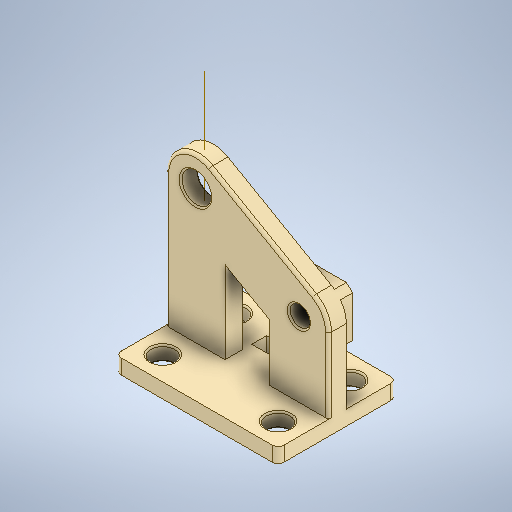
# Autodesk Inventor part: Steering Mounting Plate
Saved by Autodesk Inventor 2025.2 (Build 292293000, 293)
## iProperties
Created: 2025-02-04
Part Number: Steering Mounting Plate
Material: Generic
Document SubType Name: Modeling
Designer: eason
Density: 1 g/cm^3
Appearance: Beige
Author: eason
Autodesk Inventor part; units mm, degrees
ref_plane "YZ Plane" through (0, 0, 0) normal (1, 0, 0) x (0, 1, 0)
ref_plane "XZ Plane" through (0, 0, 0) normal (0, 1, 0) x (-1, 0, 0)
ref_plane "XY Plane" through (0, 0, 0) normal (0, 0, 1) x (1, 0, 0)
sketch "Sketch1" plane through (0, 0, 0) normal (0, 0, 1) x (1, 0, 0)
  circle A0 centre (0, 0) radius 5
  line L0 (44.8948, -50) -> (-10, -50)
  line L1 (-10, -50) -> (-10, 0)
  line L2 (0, 5) -> (-5, 5) construction
  line L3 (-5, 5) -> (-5, 0) construction
  line L4 (-10, -50) -> (44.8948, -50)
  line L5 (44.8948, -45) -> (-10, -45)
  line L6 (-10, -45) -> (-10, -50)
  line L7 (0, 0) -> (34.8948, -20) construction
  circle A1 centre (34.8948, -20) radius 3.4
  arc A2 (4.9727, 8.676) -> (-10, 0) centre (0, 0) ccw
  line L8 (-24.2121, 0) -> (57.773, 0) projected
  arc A3 (44.8948, -20) -> (39.8675, -11.324) centre (34.8948, -20) ccw
  line L9 (44.8948, -20) -> (44.8948, -50)
  line L10 (4.9727, 8.676) -> (39.8675, -11.324)
  line L11 (10, -17.2576) -> (24.8948, -25.7946)
  line L12 (24.8948, -25.7946) -> (24.8948, -45)
  line L13 (10, -17.2576) -> (10, -45)
  point P0 (-10, -45)
  dimension "d2" = 10
  dimension "d5" = 5
  dimension "d7" = 5
  dimension "d47" = 40.22
  dimension "d48" = 6.8
  dimension "d50" = 25
  dimension "d51" = 20
  dimension "d53" = 45
  constraints: 27 end point, 10 tangent, 6 point on circle, 4 centre point, 4 coincident, 4 point on line, 3 perpendicular, 2 horizontal, 1 parallel
  measures "d2" diameter of A0
  measures "d5" distance between parallel lines of L1 L3
  measures "d7" distance between parallel lines of L0 L5
  measures "d47" distance of L7.start L7.end
  measures "d48" diameter of A1
  measures "d50" distance from line of L5 L7.end
  measures "d51" diameter of A3
  measures "d53" distance from line of L5 L7.start
extrude "Extrusion1" add sketch "Sketch1" along normal mid plane 6 contours L8 L10 A3 L9 L5 L12 L11 L13 L1 A0 | A0 L8 A2 L10
extrude "Extrusion2" add sketch "Sketch1" along normal mid plane 40 contours L5 L9 L0 L1
sketch "Sketch2" plane through (-10, -50, 20) normal (0, -1, 0) x (1, 0, 0)
  circle A0 centre (46.8948, -32) radius 4
  circle A1 centre (46.8948, -8) radius 4
  circle A2 centre (8, -32) radius 4
  circle A3 centre (8, -8) radius 4
  line L0 (54.8948, -40) -> (0, -40) projected
  line L1 (54.8948, 0) -> (54.8948, -40) projected
  line L2 (0, 0) -> (54.8948, 0) projected
  line L3 (0, -40) -> (0, 0) projected
  point P0 (10, -20)
  dimension "d14" = 8
  dimension "d15" = 8
  dimension "d16" = 8
  dimension "d17" = 8
  dimension "d18" = 8
  dimension "d19" = 8
  dimension "d20" = 8
  dimension "d21" = 8
  dimension "d22" = 8
  dimension "d23" = 8
  dimension "d24" = 8
  dimension "d25" = 8
  constraints: 4 centre point
  measures "d14" diameter of A0
  measures "d15" diameter of A1
  measures "d16" diameter of A2
  measures "d17" diameter of A3
  measures "d18" distance from line of L0 A0.centre
  measures "d19" distance from line of L1 A0.centre
  measures "d20" distance from line of L2 A1.centre
  measures "d21" distance from line of L1 A1.centre
  measures "d22" distance from line of L3 A3.centre
  measures "d23" distance from line of L2 A3.centre
  measures "d24" distance from line of L0 A2.centre
  measures "d25" distance from line of L3 A2.centre
extrude "Extrusion3" cut sketch "Sketch2" against normal up to surface (5 mm away) contours A0 | A1 | A2 | A3
fillet "Fillet1" radius 2 4 edges at (-10, -47.5, -20) (-10, -47.5, 20) (44.8948, -47.5, -20) (44.8948, -47.5, 20)
fillet "Fillet2" radius 1 1 edges at (-10, -22.5, 3)
fillet "Fillet3" radius 0.5 11 edges at (-5, 0, 3) (-5, 0, -3) (-6, -45, 12) (-6, -50, 12) (32.8948, -45, 12) (32.8948, -50, 12) (32.8948, -45, -12) (32.8948, -50, -12) (-6, -45, -12) (-6, -50, -12) (31.4948, -20, 3)
sketch "Sketch3" plane through (0, 0, -3) normal (0, 0, -1) x (-1, 0, 0)
  line L0 (-40.9448, -14) -> (-28.8448, -14)
  line L1 (-28.8448, -14) -> (-28.8448, -26)
  line L2 (-28.8448, -26) -> (-40.9448, -26)
  line L3 (-40.9448, -26) -> (-40.9448, -14)
  line L4 (-40.9448, -14) -> (-28.8448, -26) construction
  line L5 (-28.8448, -14) -> (-40.9448, -26) construction
  line L6 (-26.8448, -12) -> (-26.8448, -28)
  line L7 (-26.8448, -28) -> (-42.9448, -28)
  circle A0 centre (-34.8948, -20) radius 3.4
  circle A1 centre (-34.8948, -20) radius 3.4 projected
  line L8 (-42.9448, -12.0165) -> (-42.9448, -12)
  arc A2 (-39.8675, -11.324) -> (-44.8948, -20) centre (-34.8948, -20) ccw projected
  line L9 (-42.9448, -28) -> (-42.9448, -14.0673)
  arc A3 (-39.8675, -11.324) -> (-44.8948, -20) centre (-34.8948, -20) ccw projected
  line L10 (-26.8448, -12) -> (-40.8948, -12)
  point P0 (0, 0)
  dimension "d31" = 12
  dimension "d32" = 12.1
  dimension "d35" = 2
  dimension "d36" = 2
  dimension "d54" = 6.8
  dimension "d55" = 2
  dimension "d56" = 2
  constraints: 22 end point, 5 parallel, 2 point on circle, 1 centre point, 1 coincident, 1 concentric, 1 horizontal, 1 midpoint, 1 perpendicular, 1 point on line
  measures "d31" distance between parallel lines of L2 L0
  measures "d32" distance between parallel lines of L3 L1
  measures "d35" distance between parallel lines of L1 L6
  measures "d36" distance between parallel lines of L2 L7
  measures "d54" diameter of A0
  measures "d55" distance between parallel lines of L0 L10
  measures "d56" distance between parallel lines of L3 L9
extrude "Extrusion4" add sketch "Sketch3" along normal blind 4 contours L6 L7 L9 A2 L10
sketch "Sketch5" plane through (24.8948, -45, -3) normal (0, 1, 0) x (1, 0, 0)
  line L0 (0, 3) -> (-14.8948, 3)
  line L1 (-14.8948, 3) -> (-14.8948, 8)
  line L2 (-14.8948, 8) -> (0, 8)
  line L3 (0, 8) -> (0, 3)
  line L4 (18, 17) -> (-32.8948, 17) projected
  line L5 (-7.4474, 17) -> (-7.4474, -23) construction
  line L6 (18, -23) -> (-32.8948, -23) projected
  line L7 (0, 0) -> (0, -6) projected
  line L8 (-14.8948, 0) -> (-14.8948, -6) projected
  line L9 (-14.8948, 0) -> (-34.8948, 0) projected
  point P0 (-24.8948, -3)
  point P1 (-14.8948, 5.5)
  dimension "d58" = 5
  dimension "d69" = 3
  constraints: 10 end point, 3 midpoint, 2 collinear, 1 parallel, 1 point on line
  measures "d58" distance between parallel lines of L2 L0
  measures "d69" distance between parallel lines of L9 L0
extrude "Extrusion5" cut sketch "Sketch5" against normal through all
sketch "Sketch6" plane through (24.8948, -45, -6) normal (0, 0, -1) x (-1, 0, 0)
  circle A0 centre (7.4474, -2) radius 2
  line L0 (14.8948, 0) -> (0, 0) projected
  line L1 (14.8948, -5) -> (0, -5) projected
  line L2 (0, 0) -> (14.8948, 0) projected
  line L3 (7.4474, 0) -> (7.4474, -5) construction
  point P0 (24.8948, 45)
  dimension "d65" = 3
  constraints: 3 midpoint, 2 end point, 1 centre point, 1 point on line, 1 tangent
  measures "d65" distance from line of L1 A0.centre
extrude "Extrusion6" add sketch "Sketch6" along normal up to surface (5 mm away)
sketch "Sketch4" plane through (0, 0, -3) normal (0, 0, -1) x (-1, 0, 0)
  circle A0 centre (0, 0) radius 25 construction
  circle A1 centre (0, 0) radius 5 projected
  line L0 (-17.447, -47) -> (0, 0) construction
  line L1 (-10, -45) -> (-10, -50) projected
  line L2 (-10, -50) -> (-24.8948, -50) projected
  line L3 (0, -65) -> (0, 40) projected
  dimension "d57" = 50
  dimension "d66" = 7.447
  dimension "d67" = 3
  dimension "d68" = 20.366
  constraints: 2 end point, 1 centre point, 1 coincident
  measures "d57" diameter of A0
  measures "d66" distance from line of L1 L0.start
  measures "d67" distance from line of L2 L0.start
  measures "d68" angle of L3 L0
body "Solid1"
